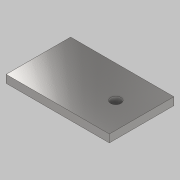
# Autodesk Inventor part: support_weldPlate
Saved by Autodesk Inventor 2021 (Build 250183000, 183)
## iProperties
Created: 2021-05-11
Part Number: support_weldPlate
Material: Steel, Galvanized
Document SubType Name: Modeling
Designer: Watchdog
Density: 7.85 g/cm^3
Appearance: Galvanized
Author: Watchdog
Autodesk Inventor part; units mm, degrees
ref_plane "YZ Plane" through (0, 0, 0) normal (1, 0, 0) x (0, 1, 0)
ref_plane "XZ Plane" through (0, 0, 0) normal (0, 1, 0) x (-1, 0, 0)
ref_plane "XY Plane" through (0, 0, 0) normal (0, 0, 1) x (1, 0, 0)
sketch "Sketch1" plane through (0, 0, 0) normal (0, 1, 0) x (-1, 0, 0)
  line L0 (40, 25) -> (-40, 25)
  line L1 (-40, 25) -> (-40, -25)
  line L2 (-40, -25) -> (40, -25)
  line L3 (40, -25) -> (40, 25)
  point P0 (0, 0)
  dimension "d0" = 50
  dimension "d1" = 40
  dimension "d2" = 80
  dimension "d3" = 25
  constraints: 8 end point, 2 parallel, 1 horizontal, 1 perpendicular
  measures "d0" distance of L2.end L0.start
  measures "d1" distance from line of point (0, 0) L3
  measures "d2" distance of L1.end L2.end
  measures "d3" distance from line of point (0, 0) L0
extrude "base" add sketch "Sketch1" along normal blind 6
sketch "Sketch2" plane through (0, 6, 0) normal (0, 1, 0) x (1, 0, 0)
  point P0 (0, 0)
  point P1 (20, 0)
  dimension "d6" = 20
  dimension "d7" = 0
  measures "d6" distance of point (0, 0) point (20, 0)
  measures "d7" vertical distance of point (0, 0) point (20, 0)
hole "mountingHole" at (20, 6, 0) direction (0, -1, 0) diameter 8 end through all
equation "\"d1\" = 0.5 * d2"
equation "\"d3\" = 0.5 * d0"
body "Solid1"
